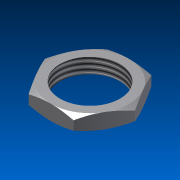
# Autodesk Inventor part: M6x0.5 Hex Nut
Saved by Autodesk Inventor 2011 SP1 (Build 150282100, 282)
## iProperties
Created: 2011-11-07
Part Number: M6x0.5 Hex Nut
Document SubType Name: Modeling
Designer: sdarley
Density: 1 g/cm^3
Author: sdarley
Autodesk Inventor part; units mm, degrees
ref_plane "YZ Plane" through (0, 0, 0) normal (1, 0, 0) x (0, 1, 0)
ref_plane "XZ Plane" through (0, 0, 0) normal (0, 1, 0) x (-1, 0, 0)
ref_plane "XY Plane" through (0, 0, 0) normal (0, 0, 1) x (1, 0, 0)
sketch "Sketch1" plane through (0, 0, 0) normal (0, 0, 1) x (1, 0, 0)
  circle A0 centre (0, 0) radius 3
  line L0 (-2.25, 3.8971) -> (2.25, 3.8971)
  line L1 (2.25, 3.8971) -> (4.5, 0)
  line L2 (4.5, 0) -> (2.25, -3.8971)
  line L3 (2.25, -3.8971) -> (-2.25, -3.8971)
  line L4 (-2.25, -3.8971) -> (-4.5, 0)
  line L5 (-4.5, 0) -> (-2.25, 3.8971)
  point P0 (0, 3.8971)
  dimension "d0" = 6
  dimension "d1" = 120
  dimension "d2" = 120
  dimension "d5" = 4.5
  dimension "d6" = 4.5
  dimension "d7" = 4.5
  dimension "d17" = 4.5
  dimension "d18" = 4.5
  dimension "d19" = 4.5
  dimension "d20" = 7.7942
  dimension "d21" = 3.8971
  constraints: 12 end point, 3 parallel, 1 centre point, 1 coincident, 1 horizontal, 1 midpoint, 1 vertical alignment
  measures "d0" diameter of A0
  measures "d1" angle of L0 L1
  measures "d2" angle of L1 L2
  measures "d5" distance of L0.start L0.end
  measures "d6" distance of L4.end L0.start
  measures "d7" distance of L0.end L1.end
  measures "d17" distance of L1.end L2.end
  measures "d18" distance of L2.end L3.end
  measures "d19" distance of L3.end L4.end
  measures "d20" distance between parallel lines of L0 L3
  measures "d21" distance from line of point (0, 0) L0
extrude "Extrusion1" add sketch "Sketch1" along normal blind 1.5
thread "Thread1" size "M6x0.5" class "6H" standard "ISO Metric profile" full length
sketch "Sketch2" plane through (0, 0, 0) normal (0, 1, 0) x (-1, 0, 0)
  line L0 (-4.5, 0) -> (-4.5, 1.5) projected
  line L1 (-2.25, 1.5) -> (-4.5, 1.5) projected
  line L2 (-2.25, 0) -> (-4.5, 0) projected
  line L3 (-4.5, 1.2) -> (-3.9, 1.5)
  line L4 (-4.5, 0.3) -> (-3.9, 0)
  line L5 (0, -0.3) -> (0, 1.8) projected
  line L6 (-4.9884, 1.5) -> (-4.9884, 0.9558)
  line L7 (-4.5, 1.2) -> (-4.9884, 0.9558)
  line L8 (-4.5, 1.5) -> (-4.9884, 1.5)
  line L9 (-4.9884, 0.5442) -> (-4.9884, 0)
  line L10 (-4.9884, 0) -> (-4.5, 0)
  line L11 (-4.5, 0.3) -> (-4.9884, 0.5442)
  point P0 (0, 0)
  dimension "d12" = 0.3
  dimension "d13" = 0.3
  dimension "d14" = 0.6
  dimension "d15" = 0.6
  constraints: 16 end point, 4 point on line, 3 collinear, 2 perpendicular, 1 parallel
  measures "d12" distance from line of L2 L4.start
  measures "d13" distance from line of L3.start L1
  measures "d14" distance from line of L3.end L0
  measures "d15" distance from line of L4.end L0
revolve "Revolution1" cut sketch "Sketch2" angle 360 about axis through (0, 0, -10) along (0, 0, 1)
equation "\"d6\" = d5"
equation "\"d7\" = d5"
equation "\"d17\" = d5"
equation "\"d21\" = 0.5 * d20"
equation "\"d13\" = d12"
equation "\"d15\" = d14"
body "Solid1"
